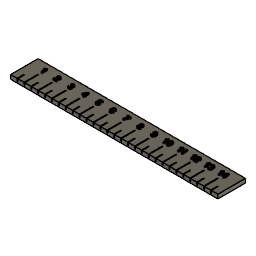
ruler (Autodesk Fusion 360 design; units mm, degrees)
part number: 2025-12-18-16-02-23-453
Autodesk Fusion 360 part; units mm, degrees
note: some values were not read from the file. Set by a fixed rule: which face or edge a step refers to.
sketch "Sketch1" plane through (0, 0, 0) normal (0, 0, 1) x (1, 0, 0)
  line L0 (0, 0) -> (150, 0)
  line L1 (150, 0) -> (150, 20)
  line L2 (150, 20) -> (0, 20)
  line L3 (0, 20) -> (0, 0)
  constraint horizontal L0
  constraint vertical L1
  constraint horizontal L2
  constraint vertical L3
  constraint coincident L0.start L3.end
extrude "Extrude1" add sketch "Sketch1" along normal blind 3
sketch "Sketch2" plane through (0, 0, 3) normal (0, 0, 1) x (-1, 0, 0)
  line L0 (0, -20) -> (0, 0)
  line L1 (0, 0) -> (-150, 0)
  line L2 (-150, 0) -> (-150, -20)
  line L3 (-150, -20) -> (0, -20)
  line L4 (0, 0) -> (-5, 0)
  line L5 (-10, 0) -> (-15, 0)
  line L6 (-20, 0) -> (-25, 0)
  line L7 (-30, 0) -> (-35, 0)
  line L8 (-40, 0) -> (-45, 0)
  line L9 (-50, 0) -> (-55, 0)
  line L10 (-60, 0) -> (-65, 0)
  line L11 (-70, 0) -> (-75, 0)
  line L12 (-80, 0) -> (-85, 0)
  line L13 (-90, 0) -> (-95, 0)
  line L14 (-100, 0) -> (-105, 0)
  line L15 (-110, 0) -> (-115, 0)
  line L16 (-120, 0) -> (-125, 0)
  line L17 (-130, 0) -> (-135, 0)
  line L18 (-140, 0) -> (-145, 0)
  line L19 (-145, 0) -> (-150, 0)
  line L20 (-135, 0) -> (-140, 0)
  line L21 (-125, 0) -> (-130, 0)
  line L22 (-115, 0) -> (-120, 0)
  line L23 (-105, 0) -> (-110, 0)
  line L24 (-100, 0) -> (-95, 0)
  line L25 (-90, 0) -> (-85, 0)
  line L26 (-75, 0) -> (-80, 0)
  line L27 (-70, 0) -> (-65, 0)
  line L28 (-55, 0) -> (-60, 0)
  line L29 (-45, 0) -> (-50, 0)
  line L30 (-35, 0) -> (-40, 0)
  line L31 (-25, 0) -> (-30, 0)
  line L32 (-15, 0) -> (-20, 0)
  line L33 (-5, 0) -> (-10, 0)
  line L34 (-5, 0) -> (-4.8, 0)
  line L35 (-4.8, 0) -> (-4.8, -5)
  line L36 (-4.8, -5) -> (-5, -5)
  line L37 (-5, -5) -> (-5, 0)
  line L38 (-5, 0) -> (-5.2, 0)
  line L39 (-5.2, 0) -> (-5.2, -5)
  line L40 (-5.2, -5) -> (-5, -5)
  line L41 (-5, -5) -> (-5, 0)
  constraint coincident L0.end L1.start
  constraint coincident L1 L4.end
  constraint coincident L1 L5.start
  constraint coincident L1 L5.end
  constraint coincident L1 L6.start
  constraint coincident L1 L6.end
  constraint coincident L1 L7.start
  constraint coincident L1 L7.end
  constraint coincident L1 L8.start
  constraint coincident L1 L8.end
  constraint coincident L1 L9.start
  constraint coincident L1 L9.end
  constraint coincident L1 L10.start
  constraint coincident L1 L10.end
  constraint coincident L1 L11.start
  constraint midpoint L1 L11.end
  constraint coincident L1 L12.start
  constraint coincident L1 L12.end
  constraint coincident L1 L13.start
  constraint coincident L1 L13.end
  constraint coincident L1 L14.start
  constraint coincident L1 L14.end
  constraint coincident L1 L15.start
  constraint coincident L1 L15.end
  constraint coincident L1 L16.start
  constraint coincident L1 L16.end
  constraint coincident L1 L17.start
  constraint coincident L1 L17.end
  constraint coincident L1 L18.start
  constraint coincident L1 L18.end
  constraint coincident L1.end L2.start
  constraint horizontal L34
  constraint vertical L35
  constraint horizontal L36
  constraint vertical L37
  constraint horizontal L38
  constraint vertical L39
  constraint horizontal L40
  constraint vertical L41
extrude "Extrude2" cut sketch "Sketch2" against normal blind 2 contours L1 L4 L34 L35 L36 L37 L41 | L1 L33 L37 L38 L39 L40 L41
pattern_linear "R-Pattern1" count 29 spacing 5 along (1, 0, 0) of "Extrude2"
extrude "Extrude3" cut 1 faces at (10.0667, 5, 2.3333) along direction (0, 1, 0) blind 5
pattern_linear "R-Pattern2" count 14 spacing 10 along (1, 0, 0) of "Extrude3"
sketch "Sketch3" plane through (0, 0, 3) normal (0, 0, 1) x (-1, 0, 0)
  line L0 (-140.2, -10) -> (-140.2, 0)
  line L1 (-140.2, 0) -> (-144.8, 0)
  line L2 (-144.8, 0) -> (-144.8, -5)
  line L3 (-144.8, -5) -> (-145.2, -5)
  line L4 (-145.2, -5) -> (-145.2, 0)
  line L5 (-145.2, 0) -> (-150, 0)
  line L6 (-150, 0) -> (-150, -20)
  line L7 (-150, -20) -> (0, -20)
  line L8 (0, -20) -> (0, 0)
  line L9 (0, 0) -> (-4.8, 0)
  line L10 (-4.8, 0) -> (-4.8, -5)
  line L11 (-4.8, -5) -> (-5.2, -5)
  line L12 (-5.2, -5) -> (-5.2, 0)
  line L13 (-5.2, 0) -> (-9.8, 0)
  line L14 (-9.8, 0) -> (-9.8, -10)
  line L15 (-9.8, -10) -> (-10.2, -10)
  line L16 (-10.2, -10) -> (-10.2, 0)
  line L17 (-10.2, 0) -> (-14.8, 0)
  line L18 (-14.8, 0) -> (-14.8, -5)
  line L19 (-14.8, -5) -> (-15.2, -5)
  line L20 (-15.2, -5) -> (-15.2, 0)
  line L21 (-15.2, 0) -> (-19.8, 0)
  line L22 (-19.8, 0) -> (-19.8, -10)
  line L23 (-19.8, -10) -> (-20.2, -10)
  line L24 (-20.2, -10) -> (-20.2, 0)
  line L25 (-20.2, 0) -> (-24.8, 0)
  line L26 (-24.8, 0) -> (-24.8, -5)
  line L27 (-24.8, -5) -> (-25.2, -5)
  line L28 (-25.2, -5) -> (-25.2, 0)
  line L29 (-25.2, 0) -> (-29.8, 0)
  line L30 (-29.8, 0) -> (-29.8, -10)
  line L31 (-29.8, -10) -> (-30.2, -10)
  line L32 (-30.2, -10) -> (-30.2, 0)
  line L33 (-30.2, 0) -> (-34.8, 0)
  line L34 (-34.8, 0) -> (-34.8, -5)
  line L35 (-34.8, -5) -> (-35.2, -5)
  line L36 (-35.2, -5) -> (-35.2, 0)
  line L37 (-35.2, 0) -> (-39.8, 0)
  line L38 (-39.8, 0) -> (-39.8, -10)
  line L39 (-39.8, -10) -> (-40.2, -10)
  line L40 (-40.2, -10) -> (-40.2, 0)
  line L41 (-40.2, 0) -> (-44.8, 0)
  line L42 (-44.8, 0) -> (-44.8, -5)
  line L43 (-44.8, -5) -> (-45.2, -5)
  line L44 (-45.2, -5) -> (-45.2, 0)
  line L45 (-45.2, 0) -> (-49.8, 0)
  line L46 (-49.8, 0) -> (-49.8, -10)
  line L47 (-49.8, -10) -> (-50.2, -10)
  line L48 (-50.2, -10) -> (-50.2, 0)
  line L49 (-50.2, 0) -> (-54.8, 0)
  line L50 (-54.8, 0) -> (-54.8, -5)
  line L51 (-54.8, -5) -> (-55.2, -5)
  line L52 (-55.2, -5) -> (-55.2, 0)
  line L53 (-55.2, 0) -> (-59.8, 0)
  line L54 (-59.8, 0) -> (-59.8, -10)
  line L55 (-59.8, -10) -> (-60.2, -10)
  line L56 (-60.2, -10) -> (-60.2, 0)
  line L57 (-60.2, 0) -> (-64.8, 0)
  line L58 (-64.8, 0) -> (-64.8, -5)
  line L59 (-64.8, -5) -> (-65.2, -5)
  line L60 (-65.2, -5) -> (-65.2, 0)
  line L61 (-65.2, 0) -> (-69.8, 0)
  line L62 (-69.8, 0) -> (-69.8, -10)
  line L63 (-69.8, -10) -> (-70.2, -10)
  line L64 (-70.2, -10) -> (-70.2, 0)
  line L65 (-70.2, 0) -> (-74.8, 0)
  line L66 (-74.8, 0) -> (-74.8, -5)
  line L67 (-74.8, -5) -> (-75.2, -5)
  line L68 (-75.2, -5) -> (-75.2, 0)
  line L69 (-75.2, 0) -> (-79.8, 0)
  line L70 (-79.8, 0) -> (-79.8, -10)
  line L71 (-79.8, -10) -> (-80.2, -10)
  line L72 (-80.2, -10) -> (-80.2, 0)
  line L73 (-80.2, 0) -> (-84.8, 0)
  line L74 (-84.8, 0) -> (-84.8, -5)
  line L75 (-84.8, -5) -> (-85.2, -5)
  line L76 (-85.2, -5) -> (-85.2, 0)
  line L77 (-85.2, 0) -> (-89.8, 0)
  line L78 (-89.8, 0) -> (-89.8, -10)
  line L79 (-89.8, -10) -> (-90.2, -10)
  line L80 (-90.2, -10) -> (-90.2, 0)
  line L81 (-90.2, 0) -> (-94.8, 0)
  line L82 (-94.8, 0) -> (-94.8, -5)
  line L83 (-94.8, -5) -> (-95.2, -5)
  line L84 (-95.2, -5) -> (-95.2, 0)
  line L85 (-95.2, 0) -> (-99.8, 0)
  line L86 (-99.8, 0) -> (-99.8, -10)
  line L87 (-99.8, -10) -> (-100.2, -10)
  line L88 (-100.2, -10) -> (-100.2, 0)
  line L89 (-100.2, 0) -> (-104.8, 0)
  line L90 (-104.8, 0) -> (-104.8, -5)
  line L91 (-104.8, -5) -> (-105.2, -5)
  line L92 (-105.2, -5) -> (-105.2, 0)
  line L93 (-105.2, 0) -> (-109.8, 0)
  line L94 (-109.8, 0) -> (-109.8, -10)
  line L95 (-109.8, -10) -> (-110.2, -10)
  line L96 (-110.2, -10) -> (-110.2, 0)
  line L97 (-110.2, 0) -> (-114.8, 0)
  line L98 (-114.8, 0) -> (-114.8, -5)
  line L99 (-114.8, -5) -> (-115.2, -5)
  line L100 (-115.2, -5) -> (-115.2, 0)
  line L101 (-115.2, 0) -> (-119.8, 0)
  line L102 (-119.8, 0) -> (-119.8, -10)
  line L103 (-119.8, -10) -> (-120.2, -10)
  line L104 (-120.2, -10) -> (-120.2, 0)
  line L105 (-120.2, 0) -> (-124.8, 0)
  line L106 (-124.8, 0) -> (-124.8, -5)
  line L107 (-124.8, -5) -> (-125.2, -5)
  line L108 (-125.2, -5) -> (-125.2, 0)
  line L109 (-125.2, 0) -> (-129.8, 0)
  line L110 (-129.8, 0) -> (-129.8, -10)
  line L111 (-129.8, -10) -> (-130.2, -10)
  line L112 (-130.2, -10) -> (-130.2, 0)
  line L113 (-130.2, 0) -> (-134.8, 0)
  line L114 (-134.8, 0) -> (-134.8, -5)
  line L115 (-134.8, -5) -> (-135.2, -5)
  line L116 (-135.2, -5) -> (-135.2, 0)
  line L117 (-135.2, 0) -> (-139.8, 0)
  line L118 (-139.8, 0) -> (-139.8, -10)
  line L119 (-139.8, -10) -> (-140.2, -10)
  line L120 (-12.5, -11) -> (-7.5, -11)
  line L121 (-7.5, -11) -> (-7.5, -17)
  line L122 (-7.5, -17) -> (-12.5, -17)
  line L123 (-12.5, -17) -> (-12.5, -11)
  line L124 (-17.5, -17) -> (-22.5, -17)
  line L125 (-17.5, -11) -> (-17.5, -17)
  line L126 (-22.5, -11) -> (-17.5, -11)
  line L127 (-22.5, -17) -> (-22.5, -11)
  line L128 (-27.5, -17) -> (-32.5, -17)
  line L129 (-27.5, -11) -> (-27.5, -17)
  line L130 (-32.5, -11) -> (-27.5, -11)
  line L131 (-32.5, -17) -> (-32.5, -11)
  line L132 (-37.5, -17) -> (-42.5, -17)
  line L133 (-37.5, -11) -> (-37.5, -17)
  line L134 (-42.5, -11) -> (-37.5, -11)
  line L135 (-42.5, -17) -> (-42.5, -11)
  line L136 (-47.5, -17) -> (-52.5, -17)
  line L137 (-47.5, -11) -> (-47.5, -17)
  line L138 (-52.5, -11) -> (-47.5, -11)
  line L139 (-52.5, -17) -> (-52.5, -11)
  line L140 (-57.5, -17) -> (-62.5, -17)
  line L141 (-57.5, -11) -> (-57.5, -17)
  line L142 (-62.5, -11) -> (-57.5, -11)
  line L143 (-62.5, -17) -> (-62.5, -11)
  line L144 (-67.5, -17) -> (-72.5, -17)
  line L145 (-67.5, -11) -> (-67.5, -17)
  line L146 (-72.5, -11) -> (-67.5, -11)
  line L147 (-72.5, -17) -> (-72.5, -11)
  line L148 (-77.5, -17) -> (-82.5, -17)
  line L149 (-77.5, -11) -> (-77.5, -17)
  line L150 (-82.5, -11) -> (-77.5, -11)
  line L151 (-82.5, -17) -> (-82.5, -11)
  line L152 (-87.5, -17) -> (-92.5, -17)
  line L153 (-87.5, -11) -> (-87.5, -17)
  line L154 (-92.5, -11) -> (-87.5, -11)
  line L155 (-92.5, -17) -> (-92.5, -11)
  line L156 (-97.5, -17) -> (-102.5, -17)
  line L157 (-97.5, -11) -> (-97.5, -17)
  line L158 (-102.5, -11) -> (-97.5, -11)
  line L159 (-102.5, -17) -> (-102.5, -11)
  line L160 (-107.5, -17) -> (-112.5, -17)
  line L161 (-107.5, -11) -> (-107.5, -17)
  line L162 (-112.5, -11) -> (-107.5, -11)
  line L163 (-112.5, -17) -> (-112.5, -11)
  line L164 (-117.5, -17) -> (-122.5, -17)
  line L165 (-117.5, -11) -> (-117.5, -17)
  line L166 (-122.5, -11) -> (-117.5, -11)
  line L167 (-122.5, -17) -> (-122.5, -11)
  line L168 (-127.5, -17) -> (-132.5, -17)
  line L169 (-127.5, -11) -> (-127.5, -17)
  line L170 (-132.5, -11) -> (-127.5, -11)
  line L171 (-132.5, -17) -> (-132.5, -11)
  line L172 (-137.5, -17) -> (-142.5, -17)
  line L173 (-137.5, -11) -> (-137.5, -17)
  line L174 (-142.5, -11) -> (-137.5, -11)
  line L175 (-142.5, -17) -> (-142.5, -11)
  line L176 (-7.5, -11) -> (-12.5, -11) construction
  line L177 (-12.5, -11) -> (-12.5, -17) construction
  line L178 (-12.5, -17) -> (-7.5, -17) construction
  line L179 (-7.5, -17) -> (-7.5, -11) construction
  line L180 (-17.5, -11) -> (-22.5, -11) construction
  line L181 (-22.5, -11) -> (-22.5, -17) construction
  line L182 (-22.5, -17) -> (-17.5, -17) construction
  line L183 (-17.5, -17) -> (-17.5, -11) construction
  line L184 (-27.5, -11) -> (-32.5, -11) construction
  line L185 (-32.5, -11) -> (-32.5, -17) construction
  line L186 (-32.5, -17) -> (-27.5, -17) construction
  line L187 (-27.5, -17) -> (-27.5, -11) construction
  line L188 (-37.5, -11) -> (-42.5, -11) construction
  line L189 (-42.5, -11) -> (-42.5, -17) construction
  line L190 (-42.5, -17) -> (-37.5, -17) construction
  line L191 (-37.5, -17) -> (-37.5, -11) construction
  line L192 (-47.5, -11) -> (-52.5, -11) construction
  line L193 (-52.5, -11) -> (-52.5, -17) construction
  line L194 (-52.5, -17) -> (-47.5, -17) construction
  line L195 (-47.5, -17) -> (-47.5, -11) construction
  line L196 (-57.5, -11) -> (-62.5, -11) construction
  line L197 (-62.5, -11) -> (-62.5, -17) construction
  line L198 (-62.5, -17) -> (-57.5, -17) construction
  line L199 (-57.5, -17) -> (-57.5, -11) construction
  line L200 (-67.5, -11) -> (-72.5, -11) construction
  line L201 (-72.5, -11) -> (-72.5, -17) construction
  line L202 (-72.5, -17) -> (-67.5, -17) construction
  line L203 (-67.5, -17) -> (-67.5, -11) construction
  line L204 (-77.5, -11) -> (-82.5, -11) construction
  line L205 (-82.5, -11) -> (-82.5, -17) construction
  line L206 (-82.5, -17) -> (-77.5, -17) construction
  line L207 (-77.5, -17) -> (-77.5, -11) construction
  line L208 (-87.5, -11) -> (-92.5, -11) construction
  line L209 (-92.5, -11) -> (-92.5, -17) construction
  line L210 (-92.5, -17) -> (-87.5, -17) construction
  line L211 (-87.5, -17) -> (-87.5, -11) construction
  line L212 (-97.5, -11) -> (-102.5, -11) construction
  line L213 (-102.5, -11) -> (-102.5, -17) construction
  line L214 (-102.5, -17) -> (-97.5, -17) construction
  line L215 (-97.5, -17) -> (-97.5, -11) construction
  line L216 (-107.5, -11) -> (-112.5, -11) construction
  line L217 (-112.5, -11) -> (-112.5, -17) construction
  line L218 (-112.5, -17) -> (-107.5, -17) construction
  line L219 (-107.5, -17) -> (-107.5, -11) construction
  line L220 (-117.5, -11) -> (-122.5, -11) construction
  line L221 (-122.5, -11) -> (-122.5, -17) construction
  line L222 (-122.5, -17) -> (-117.5, -17) construction
  line L223 (-117.5, -17) -> (-117.5, -11) construction
  line L224 (-127.5, -11) -> (-132.5, -11) construction
  line L225 (-132.5, -11) -> (-132.5, -17) construction
  line L226 (-132.5, -17) -> (-127.5, -17) construction
  line L227 (-127.5, -17) -> (-127.5, -11) construction
  line L228 (-137.5, -11) -> (-142.5, -11) construction
  line L229 (-142.5, -11) -> (-142.5, -17) construction
  line L230 (-142.5, -17) -> (-137.5, -17) construction
  line L231 (-137.5, -17) -> (-137.5, -11) construction
  dimension "d17" = -10
  dimension "d18" = 0
  dimension "d19" = 4
  dimension "d21" = 4
  dimension "d23" = 4
  dimension "d25" = 4
  dimension "d27" = 4
  dimension "d29" = 4
  dimension "d31" = 4
  dimension "d33" = 4
  dimension "d35" = 4
  dimension "d37" = 4
  dimension "d38" = 0
  dimension "d39" = 4
  dimension "d40" = 0
  dimension "d41" = 4
  dimension "d42" = 0
  dimension "d43" = 4
  dimension "d44" = 0
  dimension "d45" = 4
  dimension "d46" = 0
  text T0 "1" font "Arial" height 4 align centre middle in box 5 x 6 at (-7.5, -11) x (-1, 0) y (0, -1) spacing 1 kerned
  text T1 "2" font "Arial" height 4 align centre middle in box 5 x 6 at (-17.5, -11) x (-1, 0) y (0, -1) spacing 1 kerned
  text T2 "3" font "Arial" height 4 align centre middle in box 5 x 6 at (-27.5, -11) x (-1, 0) y (0, -1) spacing 1 kerned
  text T3 "4" font "Arial" height 4 align centre middle in box 5 x 6 at (-37.5, -11) x (-1, 0) y (0, -1) spacing 1 kerned
  text T4 "5" font "Arial" height 4 align centre middle in box 5 x 6 at (-47.5, -11) x (-1, 0) y (0, -1) spacing 1 kerned
  text T5 "6" font "Arial" height 4 align centre middle in box 5 x 6 at (-57.5, -11) x (-1, 0) y (0, -1) spacing 1 kerned
  text T6 "7" font "Arial" height 4 align centre middle in box 5 x 6 at (-67.5, -11) x (-1, 0) y (0, -1) spacing 1 kerned
  text T7 "8" font "Arial" height 4 align centre middle in box 5 x 6 at (-77.5, -11) x (-1, 0) y (0, -1) spacing 1 kerned
  text T8 "9" font "Arial" height 4 align centre middle in box 5 x 6 at (-87.5, -11) x (-1, 0) y (0, -1) spacing 1 kerned
  text T9 "10" font "Arial" height 4 align centre middle in box 5 x 6 at (-97.5, -11) x (-1, 0) y (0, -1) spacing 1 kerned
  text T10 "11" font "Arial" height 4 align centre middle in box 5 x 6 at (-107.5, -11) x (-1, 0) y (0, -1) spacing 1 kerned
  text T11 "12" font "Arial" height 4 align centre middle in box 5 x 6 at (-117.5, -11) x (-1, 0) y (0, -1) spacing 1 kerned
  text T12 "13" font "Arial" height 4 align centre middle in box 5 x 6 at (-127.5, -11) x (-1, 0) y (0, -1) spacing 1 kerned
  text T13 "14" font "Arial" height 4 align centre middle in box 5 x 6 at (-137.5, -11) x (-1, 0) y (0, -1) spacing 1 kerned
  constraint horizontal L120
  constraint perpendicular L120 L121
  constraint perpendicular L121 L122
  constraint perpendicular L120 L123
  constraint coincident L121.end
  constraint coincident L120.start
  constraint coincident L126.start
  constraint coincident L124.start
  constraint coincident L130.start
  constraint coincident L128.start
  constraint coincident L134.start
  constraint coincident L132.start
  constraint coincident L138.start
  constraint coincident L136.start
  constraint coincident L142.start
  constraint coincident L140.start
  constraint coincident L146.start
  constraint coincident L144.start
  constraint coincident L150.start
  constraint coincident L148.start
  constraint coincident L154.start
  constraint coincident L152.start
  constraint coincident L158.start
  constraint coincident L156.start
  constraint coincident L162.start
  constraint coincident L160.start
  constraint coincident L166.start
  constraint coincident L164.start
  constraint coincident L170.start
  constraint coincident L168.start
  constraint coincident L174.start
  constraint coincident L172.start
extrude "Extrude4" add sketch "Sketch3" along normal blind 1 text T0 T1 T2 T3 T4 T5 T6 T7 T8 T9 T10 T11 T12 T13
sketch "Sketch4" plane through (0, 0, 0) normal (0, 0, -1) x (1, 0, 0)
  line L0 (0, 0) -> (0, -20)
  line L1 (0, -20) -> (150, -20)
  line L2 (150, -20) -> (150, 0)
  line L3 (150, 0) -> (0, 0)
  line L4 (150, 0) -> (0, 0) construction
  line L5 (0, 0) -> (0, -20) construction
  line L6 (0, -20) -> (150, -20) construction
  line L7 (150, -20) -> (150, 0) construction
  dimension "d49" = 10
  text T0 "Tejaji" font "Arial" height 10 align centre middle in box 150 x 20 at (150, 0) x (-1, 0) y (0, -1) spacing 1 kerned
  constraint coincident L2.end
  constraint coincident L0.end
extrude "Extrude5" cut sketch "Sketch4" against normal blind 1 text T0
equation "d3 = 0 mm - 2 mm"
equation "d20 = 1"
equation "d22 = 2"
equation "d24 = 3"
equation "d26 = 4"
equation "d28 = 5"
equation "d30 = 6"
equation "d32 = 7"
equation "d34 = 8"
equation "d36 = 9"
equation "d50 = 'Tejaji'"
